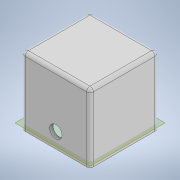
# Autodesk Inventor part: box
Saved by Autodesk Inventor 2020 (Build 240168000, 168)
## iProperties
Created: 2022-08-25
Part Number: box
Material: Типовые
Document SubType Name: Modeling
Designer: zigma
Density: 1 g/cm^3
Appearance: По умолчанию
Author: zigma
Autodesk Inventor part; units mm, degrees
ref_plane "YZ Plane" through (0, 0, 0) normal (1, 0, 0) x (0, 1, 0)
ref_plane "XZ Plane" through (0, 0, 0) normal (0, 1, 0) x (-1, 0, 0)
ref_plane "XY Plane" through (0, 0, 0) normal (0, 0, 1) x (1, 0, 0)
sketch "Эскиз1" plane through (0, 0, 0) normal (0, 1, 0) x (-1, 0, 0)
  line L0 (0, 0) -> (55, 0)
  line L1 (55, 0) -> (55, -55)
  line L2 (55, -55) -> (0, -55)
  line L3 (0, -55) -> (0, 0)
  line L4 (-3, -58) -> (58, -58)
  line L5 (58, -58) -> (58, 3)
  line L6 (58, 3) -> (-3, 3)
  line L7 (-3, 3) -> (-3, -58)
  dimension "d0" = 55
  dimension "d1" = 55
  dimension "d2" = 3
  constraints: 16 end point, 4 parallel, 2 perpendicular, 1 horizontal, 3 other
  measures "d0" distance of L1.end L2.end
  measures "d1" distance of L0.end L1.end
  measures "d2" distance between parallel lines of L2 L4
extrude "Выдавливание1" add sketch "Эскиз1" along normal blind 58
sketch "Эскиз2" plane through (0, 58, 0) normal (0, 1, 0) x (1, 0, 0)
  line L0 (-58, -3) -> (3, -3) projected
  line L1 (3, 58) -> (-58, 58) projected
  line L2 (-58, -3) -> (3, -3)
  line L3 (3, -3) -> (3, 58)
  line L4 (3, 58) -> (-58, 58)
  line L5 (-58, 58) -> (-58, -3)
  point P0 (0, 0)
  point P1 (3, -3)
  constraints: 8 end point, 2 parallel, 1 horizontal, 1 perpendicular
extrude "Выдавливание2" add sketch "Эскиз2" along normal blind 3
sketch "Эскиз3" plane through (0, 58, 0) normal (0, -1, 0) x (1, 0, 0)
  line L0 (3, -58) -> (-58, -58) projected
  line L1 (-58, 3) -> (3, 3) projected
  line L2 (-58, -58) -> (-58, 3) projected
  line L3 (3, 3) -> (3, -58) projected
  line L4 (-37.5, -17.5) -> (-17.5, -17.5)
  line L5 (-17.5, -17.5) -> (-17.5, -37.5)
  line L6 (-17.5, -37.5) -> (-37.5, -37.5)
  line L7 (-37.5, -37.5) -> (-37.5, -17.5)
  line L8 (-37.5, -27.5) -> (-17.5, -27.5) construction
  line L9 (-27.5, -37.5) -> (-27.5, -27.5) construction
  line L10 (-55, 0) -> (-55, -55) projected
  line L11 (-55, -27.5) -> (0, -27.5) construction
  line L12 (0, -55) -> (0, 0) projected
  line L13 (-55, -55) -> (0, -55) projected
  line L14 (-27.5, -55) -> (-27.5, -27.5) construction
  dimension "d7" = 20
  dimension "d8" = 20
  constraints: 16 end point, 8 midpoint, 2 parallel, 1 horizontal, 1 perpendicular
  measures "d7" distance of L5.end L6.end
  measures "d8" distance of L4.end L5.end
extrude "Выдавливание3" cut sketch "Эскиз3" against normal blind 1.5 contours L4 L5 L6 L7
ref_plane "РабПлоскость1" through (0, 5, 0) normal (0, -1, 0) x (1, 0, 0)
sketch "Эскиз4" plane through (0, 5, 0) normal (0, -1, 0) x (1, 0, 0)
  line L0 (0, -55) -> (0, 0)
  line L1 (-55, -27.5) -> (0, -27.5)
  line L2 (-27.5, -55) -> (-27.5, 0)
  line L3 (-55, 0) -> (-55, -55) projected
  line L4 (3, -58) -> (-58, -58) projected
  line L5 (3, 3) -> (3, -58) projected
  line L6 (-58, -58) -> (3, -58)
  line L7 (3, -58) -> (3, 3)
  line L8 (3, 3) -> (-58, 3)
  line L9 (-58, 3) -> (-58, -58)
  line L10 (-56, 1) -> (1, 1)
  line L11 (1, 1) -> (1, -56)
  line L12 (1, -56) -> (-56, -56)
  line L13 (-56, -56) -> (-56, 1)
  line L14 (-56, -56) -> (-43.5, -56)
  line L15 (-43.5, -56) -> (-43.5, -43.5)
  line L16 (-43.5, -43.5) -> (-56, -43.5)
  line L17 (-56, -43.5) -> (-56, -56)
  line L18 (-56, 1) -> (-43.5, 1)
  line L19 (-43.5, 1) -> (-43.5, -11.5)
  line L20 (-43.5, -11.5) -> (-56, -11.5)
  line L21 (-56, -11.5) -> (-56, 1)
  line L22 (1, -56) -> (-11.5, -56)
  line L23 (-11.5, -56) -> (-11.5, -43.5)
  line L24 (-11.5, -43.5) -> (1, -43.5)
  line L25 (1, -43.5) -> (1, -56)
  line L26 (-11.5, 1) -> (-11.5, -11.5)
  line L27 (1, 1) -> (-11.5, 1)
  line L28 (-11.5, -11.5) -> (1, -11.5)
  line L29 (1, -11.5) -> (1, 1)
  point P0 (-11.5, 1)
  point P1 (1, -11.5)
  point P2 (1, -43.5)
  point P3 (-11.5, -56)
  point P4 (-56, -11.5)
  point P5 (-43.5, 1)
  point P6 (-56, -43.5)
  point P7 (-43.5, -56)
  dimension "d14" = 2
  dimension "d15" = 12.5
  dimension "d16" = 12.5
  constraints: 54 end point, 9 symmetric about line, 7 parallel, 3 perpendicular, 2 horizontal, 1 midpoint, 3 other
  measures "d14" distance between parallel lines of L8 L10
  measures "d15" distance of L16.end L15.end
  measures "d16" distance of L15.end L14.end
extrude "Выдавливание4" cut sketch "Эскиз4" against normal blind 2.5 contours L24 L11 L12 L23 | L28 L26 L10 L11 | L12 L13 L16 L15 | L20 L13 L10 L19
fillet "Сопряжение1" radius 3 16 edges at (-55, 32.75, 0) (0, 32.75, 0) (0, 32.75, -55) (-55, 32.75, -55) (3, 30.5, 3) (-58, 30.5, 3) (-58, 30.5, -58) (-58, 61, -27.5) (-27.5, 61, -58) (3, 61, -27.5) (3, 30.5, -58) (-27.5, 61, 3) (-27.5, 58, -55) (-55, 58, -27.5) (-27.5, 58, 0) (0, 58, -27.5)
fillet "Сопряжение2" radius 3 4 edges at (0, 2.5, -55) (-55, 2.5, -55) (-55, 2.5, 0) (0, 2.5, 0)
sketch "Эскиз5" plane through (-55, 0, 3) normal (0, 0, 1) x (1, 0, 0)
  line L0 (55, 5) -> (55, 7.5) projected
  line L1 (0, 5) -> (0, 7.5) projected
  line L2 (55, 5) -> (0, 5)
  line L3 (27.5, 5) -> (27.5, 8) construction
  line L4 (27.5, 8) -> (27.5, 13.5) construction
  circle A0 centre (27.5, 13.5) radius 5.5
  point P0 (55, 0)
  dimension "d21" = 3
  dimension "d22" = 5.5
  constraints: 6 end point, 2 vertical, 1 coincident, 1 horizontal, 1 midpoint, 1 vertical alignment, 2 other
  measures "d21" distance of L3.start L3.end
  measures "d22" distance of L3.end L4.end
extrude "Выдавливание5" cut sketch "Эскиз5" against normal blind 3
equation "\"d16\" = d15"
